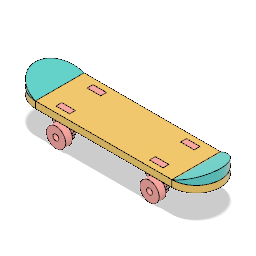
planche de skate V3 v2 (Autodesk Fusion 360 design; units mm, degrees)
Autodesk Fusion 360 part; units mm, degrees
note: some values were not read from the file. Set by a fixed rule: which face or edge a step refers to.
sketch "Esquisse1" plane through (0, 0, 0) normal (0, 1, 0) x (1, 0, 0)
  line L0 (-47.5, 12.5) -> (47.5, 12.5)
  line L1 (47.5, 12.5) -> (47.5, -12.5)
  line L2 (47.5, -12.5) -> (-47.5, -12.5)
  line L3 (-47.5, -12.5) -> (-47.5, 12.5)
  circle A0 centre (-35, 0) radius 12.5
  line L4 (0, 12.5) -> (0, -12.5) construction
  circle A1 centre (35, 0) radius 12.5
  line L5 (-27.5, 9.5) -> (-20.5, 9.5)
  line L6 (-20.5, 9.5) -> (-20.5, 6.5)
  line L7 (-20.5, 6.5) -> (-27.5, 6.5)
  line L8 (-27.5, 6.5) -> (-27.5, 9.5)
  line L9 (-47.5, 0) -> (47.5, 0) construction
  line L10 (-20.5, -6.5) -> (-27.5, -6.5)
  line L11 (-27.5, -6.5) -> (-27.5, -9.5)
  line L12 (-27.5, -9.5) -> (-20.5, -9.5)
  line L13 (-20.5, -9.5) -> (-20.5, -6.5)
  line L14 (20.5, -6.5) -> (20.5, -9.5)
  line L15 (27.5, -9.5) -> (27.5, -6.5)
  line L16 (27.5, -6.5) -> (20.5, -6.5)
  line L17 (20.5, -9.5) -> (27.5, -9.5)
  line L18 (27.5, 6.5) -> (20.5, 6.5)
  line L19 (20.5, 6.5) -> (20.5, 9.5)
  line L20 (20.5, 9.5) -> (27.5, 9.5)
  line L21 (27.5, 9.5) -> (27.5, 6.5)
  dimension "d1" = 95
  dimension "d2" = 25
  dimension "d5" = 3
  dimension "d6" = 7
  dimension "d7" = 3
  dimension "d39" = 20
  constraint horizontal L0
  constraint vertical L1
  constraint horizontal L2
  constraint vertical L3
  constraint tangent L3 A0
  constraint tangent L0 A0
  constraint tangent L2 A0
  constraint midpoint L0 L4.start
  constraint midpoint L2 L4.end
  constraint symmetric A0 L4 A1
  constraint horizontal L5
  constraint vertical L6
  constraint horizontal L7
  constraint vertical L8
  constraint midpoint L3 L9.start
  constraint midpoint L1 L9.end
  constraint symmetric L5.start L9 L11.end
  constraint symmetric L5.end L9 L12.end
  constraint symmetric L6.end L9 L10.start
  constraint symmetric L7.end L9 L10.end
  measures "d1" distance of L1.end L2.end
  measures "d2" distance of L0.start L2.end
  measures "d5" distance of L5.end L6.end
  measures "d6" distance of L6.end L7.end
  measures "d7" distance of L0 L5
  measures "d39" distance of L3 L8
extrude "Extrusion1" add sketch "Esquisse1" along normal blind 3.5 contours L0 L2 A0 A1 L5 L6 L7 L10 L12 L13 L14 L16 L17 L18 L19 L20 | A0 L5 L7 L8 L10 L11 L12 | A1 L15 L16 L17 L18 L20 L21 makes body 1
sketch "Esquisse2" plane through (0, 0, -9.5) normal (0, 0, 1) x (-1, 0, 0)
  line L0 (-31.5, 0) -> (-16.5, 0)
  circle A0 centre (-24, 7) radius 1.5
  circle A1 centre (-24, 7) radius 3.5
  line L1 (-31.5, 0) -> (-27.5, 7)
  line L2 (-24, 7) -> (-27.5, 7) construction
  line L3 (-16.5, 0) -> (-20.5, 7)
  line L4 (-20.5, 0) -> (-27.5, 0)
  line L5 (-20.5, 0) -> (-27.5, 0)
  line L6 (-20.5, -3.5) -> (-20.5, 0)
  line L7 (-27.5, -3.5) -> (-20.5, -3.5)
  line L8 (-27.5, 0) -> (-27.5, -3.5)
  point P0 (-24, 0)
  dimension "d22" = 3
  dimension "d23" = 7
  dimension "d40" = 15
  constraint concentric A0 A1
  constraint coincident A1 L1.end
  constraint coincident A0.centre A1.centre
  constraint coincident A1 L3.end
  constraint equal L1 L3
  measures "d22" diameter of A0
  measures "d23" diameter of A1
  measures "d40" distance of L0.end L0.start
extrude "Extrusion3" add sketch "Esquisse2" along normal up to surface (3 mm away) separate body makes body 2
copy_body "Copier/Coller des corps4" bodies 2 makes body 3
move_body "Déplacer4" bodies 3 to x (1, 0, 0) y (0, 1, 0) z (0, 0, 1) at (-48, 0, 0)
copy_body "Copier/Coller des corps5" bodies 2 3 makes body 4 makes body 5
move_body "Déplacer5" bodies 4 5 to x (1, 0, 0) y (0, 1, 0) z (0, 0, 1) at (0, 0, 16)
sketch "Esquisse3" plane through (0, 0, -9.5) normal (0, 0, -1) x (-1, 0, 0)
  line L0 (-20.5, -7) -> (-16.5, 0)
  circle A0 centre (-24, -7) radius 3.5
  line L1 (-31.5, 0) -> (-27.5, -7)
  circle A1 centre (-24, -7) radius 1.5
  circle A2 centre (-24, -7) radius 5
  circle A3 centre (-24, -7) radius 1.5
  line L2 (-27.5, 0) -> (-31.5, 0)
  line L3 (-16.5, 0) -> (-20.5, 0)
  line L4 (-20.5, 0) -> (-20.5, 3.5)
  line L5 (-20.5, 3.5) -> (-27.5, 3.5)
  line L6 (-27.5, 3.5) -> (-27.5, 0)
  dimension "d24" = 10
  constraint concentric A1 A2
  measures "d24" diameter of A2
extrude "Extrusion1'" add sketch "Esquisse3" along normal blind 3.5 separate body contours L0 A0 L1 A2 | A0 | L0 A0 L1 A2 makes body 6 in component "roues"
copy_body "Copier/Coller des corps6" bodies 6 makes body 7
move_body "Déplacer6" bodies 7 to x (1, 0, 0) y (0, 1, 0) z (0, 0, 1) at (-48, 0, 0)
copy_body "CutPasteBodies1" bodies 7 removing the originals makes body 8 in component "roues"
copy_body "Copier/Coller des corps7" bodies 6 8 makes body 9 makes body 10
move_body "Déplacer7" bodies 9 10 to x (1, 0, 0) y (0, 1, 0) z (0, 0, 1) at (0, 0, 22.5)
copy_body "CutPasteBodies2" bodies 9 10 removing the originals makes body 11 makes body 12 in component "roues"
ref_plane "Plan de construction1" through (0, 1.75, 0) normal (0, 0, -1) x (-1, 0, 0)
sketch "Esquisse4" plane through (0, 0, 0) normal (0, 0, 1) x (1, 0, 0)
  line L0 (47.5, 0) -> (35, 0)
  line L1 (35, 0) -> (35, 3.5)
  line L2 (47.5, 3.5) -> (35, 3.5)
  line L3 (35, 3.5) -> (35, 0)
  line L4 (47.5, 3.5) -> (47.5, 8.5)
  line L5 (47.5, 8.5) -> (35, 3.5)
  line L6 (47.5, 3.5) -> (35, 3.5)
  dimension "d50" = 5
  dimension "d51" = 12.5
  constraint coincident L2.start L4.start
  constraint perpendicular L2 L4
  constraint coincident L1.end L2.end
  measures "d50" distance of L2.start L4.end
  measures "d51" distance of L2.start L1.end
extrude "Extrusion5" add sketch "Esquisse4" along normal mid plane 40 separate body makes body 13
extrude "Extrusion6" cut sketch "Esquisse1" along normal blind 27 contours A1 L15 L16 L17 L18 L20 L21 keep common part bodies 13
sketch "Esquisse5" plane through (0, 3.5, 0) normal (0, -1, 0) x (1, 0, 0)
  arc A0 (35, -12.5) -> (35, 12.5) centre (35, 0) ccw
  line L0 (35, 12.5) -> (35, -12.5)
  line L1 (38.5, 0) -> (43.5, 0)
  line L2 (43.5, 0) -> (43.5, 2.5)
  line L3 (43.5, 2.5) -> (38.5, 2.5)
  line L4 (38.5, 2.5) -> (38.5, 0)
  line L5 (43.4108, 0) -> (-42, 0)
  line L6 (38.5, -2.5) -> (38.5, 0)
  line L7 (43.5, -2.5) -> (38.5, -2.5)
  line L8 (43.5, 0) -> (43.5, -2.5)
  dimension "d56" = 5
  dimension "d57" = 3.5
  dimension "d59" = 2.5
  constraint horizontal L1
  constraint vertical L2
  constraint horizontal L3
  constraint vertical L4
  constraint symmetric L1.start L5 L4.end
  constraint symmetric L1.end L5 L2.start
  constraint symmetric L2.end L5 L7.start
  constraint symmetric L3.end L5 L6.start
  measures "d56" distance of L1.start L1.end
  measures "d57" distance of L0 L4
  measures "d59" distance of L1.end L2.end
extrude "Extrusion7" add sketch "Esquisse5" along normal blind 3.5 contours L1 L2 L3 L4 L5 | L1 L5 L6 L7 L8 bodies 13
copy_body "Corps->Comp1" bodies 5 removing the originals makes body 14 in component "fixations"
copy_body "CutPasteBodies1'" bodies 4 removing the originals makes body 15 in component "fixations"
copy_body "CutPasteBodies2'" bodies 3 removing the originals makes body 16 in component "fixations"
copy_body "CutPasteBodies3" bodies 2 removing the originals makes body 17 in component "fixations"
copy_body "Corps->Comp2" bodies 1 removing the originals makes body 18 in component "planche"
ref_plane "Plan de construction2" through (0, 1.75, -8) normal (-1, 0, 0) x (0, -1, 0)
ref_plane "Plan de construction3" through (0, 1.75, -8) normal (1, 0, 0) x (0, 1, 0)
mirror "Symétrie miroir1" about plane through (0, 1.75, -8) normal (-1, 0, 0) of bodies 13 makes body 19
combine "Combiner1" operation cut target body 18 tool bodies 13 19 keep tools in component "planche"
fillet "Congé1" radius 0.5 4 edges at (41, 0, 2.5) (43.5, 0, 0) (41, 0, -2.5) (38.5, 0, 0) on bodies 13 19
fillet "Congé1" radius 0.5 4 edges at (-43.5, 0, 0) (-41, 0, 2.5) (-41, 0, -2.5) (-38.5, 0, 0) on bodies 13 19
copy_body "Corps->Comp3" bodies 13 removing the originals makes body 20 in component "3d prints"
copy_body "CutPasteBodies1''" bodies 19 removing the originals makes body 21 in component "3d prints"
component "roues" placed x (1, 0, 0) y (0, 1, 0) z (0, 0, 1) at (0, 0, 0)
component "fixations" placed x (1, 0, 0) y (0, 1, 0) z (0, 0, 1) at (0, 0, 0)
component "planche" placed x (1, 0, 0) y (0, 1, 0) z (0, 0, 1) at (0, 0, 0)
component "3d prints" placed x (1, 0, 0) y (0, 1, 0) z (0, 0, 1) at (0, 0, 0)
equation "d3 = ep_bois"
equation "d7 = ep_bois - 0.5 mm"
equation "hauteurtruck = 7 mm"
equation "axe = 3 mm"
equation "dia_truck = 7 mm"
equation "d22 = axe"
equation "d23 = dia_truck"
equation "d24 = dia_roue"
equation "dia_roue = 10 mm"
equation "ep_bois = 3.5 mm"
equation "d27 = ep_bois"
